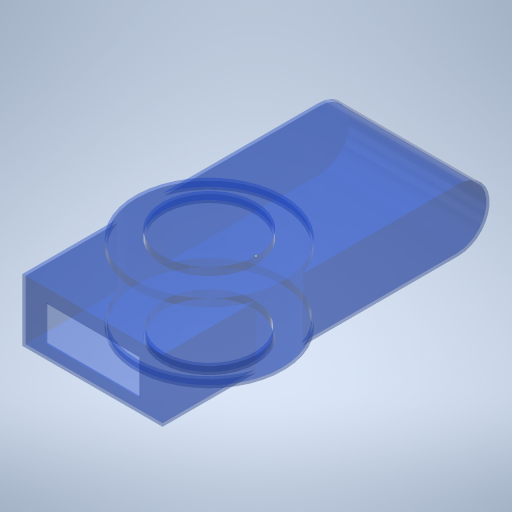
# Autodesk Inventor part: Pendrive
Saved by Autodesk Inventor 2024.2 (Build 282272000, 272)
## iProperties
Created: 2024-04-15
Part Number: Pendrive
Material: ABS Plastic
Document SubType Name: Modeling
Designer: 082220022
Density: 1.06 g/cm^3
Appearance: Clear - Blue
Mass: 0.52859 g
Surface Area: 49.9359 cm^2
Volume: 0.49867 cm^3
Author: 082220022
Autodesk Inventor part; units mm, degrees
ref_plane "YZ Plane" through (0, 0, 0) normal (1, 0, 0) x (0, 1, 0)
ref_plane "XZ Plane" through (0, 0, 0) normal (0, 1, 0) x (-1, 0, 0)
ref_plane "XY Plane" through (0, 0, 0) normal (0, 0, 1) x (1, 0, 0)
sketch "Sketch1" plane through (0, 0, 0) normal (0, 1, 0) x (-1, 0, 0)
  point P0 (0, 0)
sketch "Sketch2" plane through (0, 0, 0) normal (0, 0, 1) x (1, 0, 0)
  line L0 (-21, -9) -> (-21, 9)
  line L1 (-21, 9) -> (21, 9)
  line L2 (21, 9) -> (21, -9)
  line L3 (21, -9) -> (-21, -9)
  point P0 (0, 0)
  dimension "d0" = 42
  dimension "d1" = 18
  dimension "d2" = 21
  dimension "d3" = 9
  constraints: 8 end point, 1 horizontal, 1 parallel, 1 perpendicular, 1 vertical
  measures "d0" distance of L0.end L1.end
  measures "d1" distance of L0.start L0.end
  measures "d2" distance from line of L0 point (0, 0)
  measures "d3" distance from line of L1 point (0, 0)
extrude "Extrusion1" add sketch "Sketch2" along normal mid plane 8
fillet "Fillet1" radius 4 2 edges at (21, 0, 4) (21, 0, -4)
sketch "Sketch3" plane through (0, 0, 4) normal (0, 0, 1) x (1, 0, 0)
  circle A0 centre (-6, 0) radius 9.5
  line L0 (-21, -9) -> (-21, 9) projected
  point P0 (0, 0)
  dimension "d7" = 19
  dimension "d8" = 15
  dimension "d9" = 0
  constraints: 1 centre point
  measures "d7" diameter of A0
  measures "d8" distance from line of L0 A0.centre
  measures "d9" vertical distance of point (0, 0) A0.centre
extrude "Extrusion2" add sketch "Sketch3" along normal blind 1 and the other way blind 9
sketch "Sketch4" plane through (-6, 0, 5) normal (0, 0, 1) x (1, 0, 0)
  circle A0 centre (0, 0) radius 6
  point P0 (6, 0)
  dimension "d14" = 12
  constraints: 1 centre point
  measures "d14" diameter of A0
extrude "Extrusion3" add sketch "Sketch4" along normal blind 1 and the other way blind 11
shell "Shell1" thickness 0.2 removed faces 0
sketch "Sketch5" plane through (-21, -9, 4) normal (-1, 0, 0) x (0, 0, 1)
  line L0 (-1.75, 15) -> (-6.25, 15)
  line L1 (-6.25, 15) -> (-6.25, 3)
  line L2 (-6.25, 3) -> (-1.75, 3)
  line L3 (-1.75, 3) -> (-1.75, 15)
  line L4 (-8, 18) -> (0, 18) projected
  line L5 (0, 18) -> (0, 0) projected
  point P0 (-4, 9)
  dimension "d20" = 12
  dimension "d21" = 4.5
  dimension "d22" = 3
  dimension "d23" = 1.75
  constraints: 8 end point, 2 parallel, 1 horizontal, 1 perpendicular
  measures "d20" distance of L2.end L0.start
  measures "d21" distance of L0.start L0.end
  measures "d22" distance between parallel lines of L0 L4
  measures "d23" distance between parallel lines of L5 L3
extrude "Extrusion4" cut sketch "Sketch5" against normal blind 1
equation "\"d2\" = 0.5 * d0"
equation "\"d3\" = 0.5 * d1"
body "Solid1"
